# Autodesk Inventor part: flange_8mm
Saved by Autodesk Inventor 2021 (Build 250183000, 183)
## iProperties
Created: 2021-01-22
Part Number: flange_8mm
Material: Aluminum
Document SubType Name: Modeling
Designer: User
Density: 2.7 g/cm^3
Appearance: Semi-Polished
Author: User
Autodesk Inventor part; units mm, degrees
ref_plane "YZ Plane" through (0, 0, 0) normal (1, 0, 0) x (0, 1, 0)
ref_plane "XZ Plane" through (0, 0, 0) normal (0, 1, 0) x (-1, 0, 0)
ref_plane "XY Plane" through (0, 0, 0) normal (0, 0, 1) x (1, 0, 0)
sketch "Sketch1" plane through (0, 0, 0) normal (0, 1, 0) x (-1, 0, 0)
  circle A0 centre (0, 0) radius 16
  circle A1 centre (0, 0) radius 4
  circle A2 centre (0, 0) radius 8
  circle A3 centre (12, 0) radius 2
  circle A4 centre (0, 12) radius 2
  circle A5 centre (-12, 0) radius 2
  circle A6 centre (0, -12) radius 2
  dimension "d0" = 32
  dimension "d1" = 8
  dimension "d4" = 4
  dimension "d7" = 360
  dimension "d9" = 24
  dimension "d10" = 16
  constraints: 7 centre point, 3 coincident, 1 horizontal alignment, 9 other
  measures "d0" diameter of A0
  measures "d1" diameter of A1
  measures "d4" diameter of A3
  measures "d9" distance of A5.centre A3.centre
  measures "d10" diameter of A2
extrude "Extrusion1" add sketch "Sketch1" along normal blind 3 contours A0
extrude "Extrusion2" add sketch "Sketch1" along normal blind 13 contours A2
body "Solid1"
